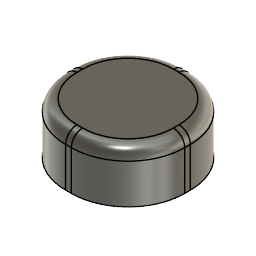
keycap (Autodesk Fusion 360 design; units mm, degrees)
Autodesk Fusion 360 part; units mm, degrees
sketch "Sketch1" plane through (0, 0, 0) normal (0, 0, 1) x (1, 0, 0)
  line L0 (-0.6, 1) -> (-0.6, 2.15)
  line L1 (-0.6, 2.15) -> (0.6, 2.15)
  line L2 (0.6, 2.15) -> (0.6, 1)
  line L3 (0.9, 0.7) -> (2.15, 0.7)
  line L4 (2.15, 0.7) -> (2.15, -0.7)
  line L5 (2.15, -0.7) -> (0.9, -0.7)
  line L6 (0.6, -1) -> (0.6, -2.15)
  line L7 (0.6, -2.15) -> (-0.6, -2.15)
  line L8 (-0.6, -2.15) -> (-0.6, -1)
  line L9 (-0.9, -0.7) -> (-2.15, -0.7)
  line L10 (-2.15, -0.7) -> (-2.15, 0.7)
  line L11 (-2.15, 0.7) -> (-0.9, 0.7)
  arc A0 (-0.9, 0.7) -> (-0.6, 1) centre (-0.9, 1) ccw
  arc A1 (0.6, 1) -> (0.9, 0.7) centre (0.9, 1) ccw
  arc A2 (-0.6, -1) -> (-0.9, -0.7) centre (-0.9, -1) ccw
  arc A3 (0.9, -0.7) -> (0.6, -1) centre (0.9, -1) ccw
  circle A4 centre (0, 0) radius 3
  point P0 (0.6, 0.7)
  dimension "d2" = 4.3
  dimension "d3" = 4.3
  dimension "d4" = 2.15
  dimension "d5" = 2.15
  dimension "d6" = 1.2
  dimension "d7" = 1.4
  dimension "d8" = 0.7
  dimension "d9" = 0.6
  dimension "d10" = 0.3
  dimension "d11" = 6
  constraint vertical L0
  constraint perpendicular L0 L1
  constraint perpendicular L1 L2
  constraint perpendicular L2 L3
  constraint perpendicular L3 L4
  constraint perpendicular L4 L5
  constraint perpendicular L3 L6
  constraint perpendicular L6 L7
  constraint perpendicular L7 L8
  constraint perpendicular L8 L9
  constraint perpendicular L7 L10
  constraint perpendicular L0 L11
  constraint tangent L0 A0
  constraint tangent L11 A0
  constraint coincident P0 L2
  constraint coincident P0 L3
  constraint tangent L2 A1
  constraint tangent L3 A1
  constraint equal A0 A1
  constraint tangent L8 A2
  constraint tangent L9 A2
  constraint equal A0 A2
  constraint tangent L5 A3
  constraint tangent L6 A3
  constraint equal A0 A3
  constraint horizontal P0 L11.end
  constraint horizontal L9.start L5.end
  constraint vertical L0.start L8.end
  constraint vertical P0 L6.start
  constraint coincident A4.centre origin
  measures "d2" distance of L4 L10
  measures "d3" distance of L1 L7
  measures "d4" distance of A4.centre L4
  measures "d5" distance of A4.centre L7
  measures "d6" distance of L0.end L1.end
  measures "d7" distance of L3.end L4.end
  measures "d8" vertical distance of A4.centre P0
  measures "d9" horizontal distance of A4.centre P0
  measures "d10" radius of A0
  measures "d11" diameter of A4
extrude "Extrude1" add sketch "Sketch1" along normal blind 7
sketch "Sketch2" plane through (0, 0, 7) normal (0, 0, 1) x (-1, 0, 0)
  line L0 (-2.15, 0.7) -> (-0.9, 0.7)
  arc A0 (-0.9, 0.7) -> (-0.6, 1) centre (-0.9, 1) ccw
  line L1 (-0.6, 1) -> (-0.6, 2.15)
  line L2 (-0.6, 2.15) -> (0.6, 2.15)
  line L3 (0.6, 2.15) -> (0.6, 1)
  arc A1 (0.6, 1) -> (0.9, 0.7) centre (0.9, 1) ccw
  line L4 (0.9, 0.7) -> (2.15, 0.7)
  line L5 (2.15, 0.7) -> (2.15, -0.7)
  line L6 (2.15, -0.7) -> (0.9, -0.7)
  arc A2 (0.9, -0.7) -> (0.6, -1) centre (0.9, -1) ccw
  line L7 (0.6, -1) -> (0.6, -2.15)
  line L8 (0.6, -2.15) -> (-0.6, -2.15)
  line L9 (-0.6, -2.15) -> (-0.6, -1)
  arc A3 (-0.6, -1) -> (-0.9, -0.7) centre (-0.9, -1) ccw
  line L10 (-0.9, -0.7) -> (-2.15, -0.7)
  line L11 (-2.15, -0.7) -> (-2.15, 0.7)
  circle A4 centre (0, 0) radius 3
  line L12 (10.5, 10.5) -> (-10.5, 10.5)
  line L13 (-10.5, 10.5) -> (-10.5, -10.5)
  line L14 (-10.5, -10.5) -> (10.5, -10.5)
  line L15 (10.5, -10.5) -> (10.5, 10.5)
  dimension "d14" = 21
  dimension "d15" = 21
  dimension "d16" = 10.5
  dimension "d17" = 10.5
  constraint horizontal L12
  constraint vertical L13
  constraint horizontal L14
  constraint vertical L15
  measures "d14" distance of L12.start L12.end
  measures "d15" distance of L12.start L14.end
  measures "d16" horizontal distance of A4.centre L12.start
  measures "d17" vertical distance of A4.centre L12.start
extrude "Extrude2" add sketch "Sketch2" along normal blind 2 contours L0 A0 L1 L2 L3 A1 L4 L5 L6 A2 L7 L8 L9 A3 L10 L11 | A4 | L12 L13 L14 L15
sketch "Sketch3" plane through (0, 0, 7) normal (0, 0, -1) x (1, 0, 0)
  line L0 (-10.5, 10.5) -> (-10.5, -10.5)
  line L1 (-10.5, -10.5) -> (10.5, -10.5)
  line L2 (10.5, -10.5) -> (10.5, 10.5)
  line L3 (10.5, 10.5) -> (-10.5, 10.5)
  circle A0 centre (0, 0) radius 3
  line L4 (10.5, -10.5) -> (-10.5, -10.5)
  line L5 (-10.5, -10.5) -> (-10.5, 10.5)
  line L6 (-10.5, 10.5) -> (10.5, 10.5)
  line L7 (10.5, 10.5) -> (10.5, -10.5)
  line L8 (-8.9, 8.9) -> (8.9, 8.9)
  line L9 (8.9, 8.9) -> (8.9, -8.9)
  line L10 (8.9, -8.9) -> (-8.9, -8.9)
  line L11 (-8.9, -8.9) -> (-8.9, 8.9)
  dimension "d20" = 1.6
  dimension "d21" = 1.6
  dimension "d22" = 1.6
  dimension "d23" = 1.6
  constraint horizontal L4
  constraint vertical L5
  constraint horizontal L6
  constraint vertical L7
  constraint coincident L0.start L3.end
  constraint coincident L1.end L2.start
  constraint horizontal L8
  constraint vertical L9
  constraint horizontal L10
  constraint vertical L11
  measures "d20" vertical distance of L1.end L9.end
  measures "d21" horizontal distance of L1.end L9.end
  measures "d22" horizontal distance of L0.end L10.end
  measures "d23" vertical distance of L0.start L8.start
extrude "Extrude3" add sketch "Sketch3" along normal blind 7 contours L0 L1 L2 L3 L4 L5 L6 L7
fillet "Fillet1" radius 3 1 faces at (0.0747, 6.9305, 7)
fillet "Fillet1" radius 8.4 4 edges at (-8.9, -8.9, 3.5) (-8.9, 8.9, 3.5) (8.9, 8.9, 3.5) (8.9, -8.9, 3.5)
fillet "Fillet1" radius 10 4 edges at (-10.5, -10.5, 4.5) (-10.5, 10.5, 4.5) (10.5, -10.5, 4.5) (10.5, 10.5, 4.5)
fillet "Fillet1" radius 2 1 faces at (3.5, 3.5, 9)
extrude "Extrude4" add 1 faces at (-0.2345, 0.2578, 7) along direction (0, 0, -1) blind 3.3
equation "d8 = ( 1.4 / 2 ) * 1 mm"
equation "d9 = ( 1.2 / 2 ) * 1 mm"
equation "d14 = 25 mm - 4 mm"
equation "d15 = 25 mm - 4 mm"
equation "d16 = ( 21 / 2 ) * 1 mm"
equation "d17 = ( 21 / 2 ) * 1 mm"
equation "d34 = 7 mm - 3.7 mm"
